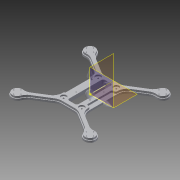
# Autodesk Inventor part: base
Saved by Autodesk Inventor 2013 (Build 170138000, 138)
## iProperties
Created: 2013-06-25
Part Number: base
Material: Aluminum 6061
Document SubType Name: Modeling
Designer: Piotr
Density: 2.71 g/cm^3
Mass: 149.971 g
Surface Area: 272.178 cm^2
Volume: 55.3399 cm^3
Author: Piotr
Autodesk Inventor part; units mm, degrees
ref_plane "YZ Plane" through (0, 0, 0) normal (1, 0, 0) x (0, 1, 0)
ref_plane "XZ Plane" through (0, 0, 0) normal (0, 1, 0) x (-1, 0, 0)
ref_plane "XY Plane" through (0, 0, 0) normal (0, 0, 1) x (1, 0, 0)
sketch "Sketch3" plane through (0, 0, 0) normal (0, 0, 1) x (1, 0, 0)
  line L0 (0, 49) -> (20.5112, 49)
  line L1 (30, 43.117) -> (30, 0)
  line L2 (30, 49) -> (80, 80) construction
  line L3 (30, 43.117) -> (72.8978, 69.7136)
  line L4 (20.5112, 49) -> (67.6284, 78.2127)
  circle A0 centre (80, 80) radius 12.5 construction
  arc A1 (72.8978, 69.7136) -> (67.6284, 78.2127) centre (80, 80) ccw
  line L5 (0, 136.0947) -> (0, -136.0947) construction
  line L6 (-136.0947, 0) -> (136.0947, 0) construction
  line L7 (0, 49) -> (-20.5112, 49)
  line L8 (-30, 43.117) -> (-30, 0)
  line L9 (-30, 43.117) -> (-72.8978, 69.7136)
  line L10 (-20.5112, 49) -> (-67.6284, 78.2127)
  arc A2 (-67.6284, 78.2127) -> (-72.8978, 69.7136) centre (-80, 80) ccw
  line L11 (0, -49) -> (20.5112, -49)
  line L12 (30, -43.117) -> (30, 0)
  line L13 (30, -43.117) -> (72.8978, -69.7136)
  line L14 (20.5112, -49) -> (67.6284, -78.2127)
  arc A3 (67.6284, -78.2127) -> (72.8978, -69.7136) centre (80, -80) ccw
  line L15 (-30, -43.117) -> (-72.8978, -69.7136)
  line L16 (-20.5112, -49) -> (-67.6284, -78.2127)
  line L17 (0, -49) -> (-20.5112, -49)
  line L18 (-30, -43.117) -> (-30, 0)
  arc A4 (-72.8978, -69.7136) -> (-67.6284, -78.2127) centre (-80, -80) ccw
  point P0 (0, 0)
  dimension "d13" = 80
  dimension "d14" = 80
  dimension "d15" = 5
  dimension "d16" = 5
  dimension "d17" = 25
  dimension "d18" = 30
  dimension "d19" = 49
  constraints: 34 end point, 17 symmetric about line, 10 point on circle, 5 centre point, 2 horizontal alignment, 2 parallel, 2 vertical alignment, 1 coincident, 1 concentric, 1 horizontal, 1 perpendicular, 3 other
  measures "d13" horizontal distance of L2.end point (0, 0)
  measures "d14" horizontal distance of point (0, 0) L2.end
  measures "d15" distance between parallel lines of L3 L2
  measures "d16" distance between parallel lines of L2 L4
  measures "d17" diameter of A0
  measures "d18" horizontal distance of point (0, 0) L2.start
  measures "d19" vertical distance of point (0, 0) L2.start
extrude "Extrusion2" add sketch "Sketch3" along normal blind 4
fillet "Fillet1" radius 20 8 edges at (30, 43.117, 2) (30, -43.117, 2) (-30, 43.117, 2) (20.5112, -49, 2) (-30, -43.117, 2) (20.5112, 49, 2) (-20.5112, 49, 2) (-20.5112, -49, 2)
fillet "Fillet2" radius 20 8 edges at (72.8978, 69.7136, 2) (-67.6284, -78.2127, 2) (-72.8978, 69.7136, 2) (67.6284, -78.2127, 2) (72.8978, -69.7136, 2) (67.6284, 78.2127, 2) (-67.6284, 78.2127, 2) (-72.8978, -69.7136, 2)
sketch "Sketch4" plane through (0, 0, 4) normal (0, 0, 1) x (1, 0, 0)
  line L0 (14.8143, 49) -> (-14.8143, 49) projected
  arc A0 (-25.3531, 52.0019) -> (-14.8143, 49) centre (-14.8143, 69) ccw projected
  line L1 (-25.3531, 52.0019) -> (-59.7157, 73.3068) projected
  arc A1 (-68.145, 83.9634) -> (-59.7157, 73.3068) centre (-49.177, 90.3048) ccw projected
  arc A2 (-68.145, 83.9634) -> (-78.2784, 67.6191) centre (-80, 80) ccw projected
  arc A3 (-64.9851, 64.8078) -> (-78.2784, 67.6191) centre (-75.5239, 47.8097) ccw projected
  line L2 (-64.9851, 64.8078) -> (-39.4612, 48.9829) projected
  arc A4 (-30, 31.9849) -> (-39.4612, 48.9829) centre (-50, 31.9849) ccw projected
  line L3 (-30, 31.9849) -> (-30, -31.9849) projected
  arc A5 (-39.4612, -48.9829) -> (-30, -31.9849) centre (-50, -31.9849) ccw projected
  line L4 (-39.4612, -48.9829) -> (-64.9851, -64.8078) projected
  arc A6 (-78.2784, -67.6191) -> (-64.9851, -64.8078) centre (-75.5239, -47.8097) ccw projected
  arc A7 (-78.2784, -67.6191) -> (-68.145, -83.9634) centre (-80, -80) ccw projected
  arc A8 (-59.7157, -73.3068) -> (-68.145, -83.9634) centre (-49.177, -90.3048) ccw projected
  line L5 (-59.7157, -73.3068) -> (-25.3531, -52.0019) projected
  arc A9 (-14.8143, -49) -> (-25.3531, -52.0019) centre (-14.8143, -69) ccw projected
  line L6 (-14.8143, -49) -> (14.8143, -49) projected
  arc A10 (25.3531, -52.0019) -> (14.8143, -49) centre (14.8143, -69) ccw projected
  line L7 (25.3531, -52.0019) -> (59.7157, -73.3068) projected
  arc A11 (68.145, -83.9634) -> (59.7157, -73.3068) centre (49.177, -90.3048) ccw projected
  arc A12 (68.145, -83.9634) -> (78.2784, -67.6191) centre (80, -80) ccw projected
  arc A13 (64.9851, -64.8078) -> (78.2784, -67.6191) centre (75.5239, -47.8097) ccw projected
  line L8 (64.9851, -64.8078) -> (39.4612, -48.9829) projected
  arc A14 (30, -31.9849) -> (39.4612, -48.9829) centre (50, -31.9849) ccw projected
  line L9 (30, -31.9849) -> (30, 31.9849) projected
  arc A15 (39.4612, 48.9829) -> (30, 31.9849) centre (50, 31.9849) ccw projected
  line L10 (39.4612, 48.9829) -> (64.9851, 64.8078) projected
  arc A16 (78.2784, 67.6191) -> (64.9851, 64.8078) centre (75.5239, 47.8097) ccw projected
  arc A17 (78.2784, 67.6191) -> (68.145, 83.9634) centre (80, 80) ccw projected
  arc A18 (59.7157, 73.3068) -> (68.145, 83.9634) centre (49.177, 90.3048) ccw projected
  line L11 (59.7157, 73.3068) -> (25.3531, 52.0019) projected
  arc A19 (14.8143, 49) -> (25.3531, 52.0019) centre (14.8143, 69) ccw projected
  line L12 (-14.8143, 47.5) -> (14.8143, 47.5)
  arc A20 (14.8143, 47.5) -> (26.1435, 50.7271) centre (14.8143, 69) ccw
  line L13 (26.1435, 50.7271) -> (60.5062, 72.0319)
  arc A21 (60.5062, 72.0319) -> (69.5676, 83.4878) centre (49.177, 90.3048) ccw
  arc A22 (78.485, 69.1048) -> (69.5676, 83.4878) centre (80, 80) ccw
  arc A23 (78.485, 69.1048) -> (64.1947, 66.0826) centre (75.5239, 47.8097) ccw
  line L14 (64.1947, 66.0826) -> (38.6708, 50.2578)
  arc A24 (38.6708, 50.2578) -> (28.5, 31.9849) centre (50, 31.9849) ccw
  line L15 (28.5, 31.9849) -> (28.5, -31.9849)
  arc A25 (28.5, -31.9849) -> (38.6708, -50.2578) centre (50, -31.9849) ccw
  line L16 (38.6708, -50.2578) -> (64.1947, -66.0826)
  arc A26 (64.1947, -66.0826) -> (78.485, -69.1048) centre (75.5239, -47.8097) ccw
  arc A27 (69.5676, -83.4878) -> (78.485, -69.1048) centre (80, -80) ccw
  arc A28 (69.5676, -83.4878) -> (60.5062, -72.0319) centre (49.177, -90.3048) ccw
  line L17 (60.5062, -72.0319) -> (26.1435, -50.7271)
  arc A29 (26.1435, -50.7271) -> (14.8143, -47.5) centre (14.8143, -69) ccw
  line L18 (14.8143, -47.5) -> (-14.8143, -47.5)
  arc A30 (-14.8143, -47.5) -> (-26.1435, -50.7271) centre (-14.8143, -69) ccw
  line L19 (-26.1435, -50.7271) -> (-60.5062, -72.0319)
  arc A31 (-60.5062, -72.0319) -> (-69.5676, -83.4878) centre (-49.177, -90.3048) ccw
  arc A32 (-78.485, -69.1048) -> (-69.5676, -83.4878) centre (-80, -80) ccw
  arc A33 (-78.485, -69.1048) -> (-64.1947, -66.0826) centre (-75.5239, -47.8097) ccw
  line L20 (-64.1947, -66.0826) -> (-38.6708, -50.2578)
  arc A34 (-38.6708, -50.2578) -> (-28.5, -31.9849) centre (-50, -31.9849) ccw
  line L21 (-28.5, -31.9849) -> (-28.5, 31.9849)
  arc A35 (-28.5, 31.9849) -> (-38.6708, 50.2578) centre (-50, 31.9849) ccw
  line L22 (-38.6708, 50.2578) -> (-64.1947, 66.0826)
  arc A36 (-64.1947, 66.0826) -> (-78.485, 69.1048) centre (-75.5239, 47.8097) ccw
  arc A37 (-69.5676, 83.4878) -> (-78.485, 69.1048) centre (-80, 80) ccw
  arc A38 (-69.5676, 83.4878) -> (-60.5062, 72.0319) centre (-49.177, 90.3048) ccw
  line L23 (-60.5062, 72.0319) -> (-26.1435, 50.7271)
  arc A39 (-26.1435, 50.7271) -> (-14.8143, 47.5) centre (-14.8143, 69) ccw
  point P0 (0, 0)
  dimension "d24" = 7
  constraints: 40 point on circle, 24 end point, 20 centre point, 31 other
  measures "d24" distance between parallel lines of L23 L22
extrude "Extrusion3" add sketch "Sketch4" along normal blind 4 contours L12 A20 L13 A21 A22 A23 L14 A24 L15 A25 L16 A26 A27 A28 L17 A29 L18 A30 L19 A31 A32 A33 L20 A34 L21 A35 L22 A36 A37 A38 L23 A39
sketch "Sketch5" plane through (0, 0, 0) normal (0, 0, -1) x (-1, 0, 0)
  line L0 (-129.5, 0) -> (129.5, 0) projected
  line L1 (0, -129.5) -> (0, 129.5) projected
  point P0 (0, 0)
  point P1 (-15.25, -15.25)
  point P2 (15.25, -15.25)
  point P3 (15.25, 15.25)
  point P4 (-15.25, 15.25)
  dimension "d28" = 30.5
  dimension "d30" = 30.5
  constraints: 2 horizontal alignment, 2 symmetric about line, 2 vertical alignment
  measures "d28" distance of point (15.25, -15.25) point (15.25, 15.25)
  measures "d30" distance of point (-15.25, 15.25) point (15.25, 15.25)
hole "Hole1" at (15.25, -15.25, 0) at (-15.25, -15.25, 0) at (-15.25, 15.25, 0) at (15.25, 15.25, 0) direction (0, 0, 1) diameter 2.1 end through all
sketch "Sketch6" plane through (0, 0, 8) normal (0, 0, 1) x (1, 0, 0)
  point P0 (0, 0)
  point P1 (-20, -38)
  dimension "d58" = 20
  dimension "d59" = 38
  measures "d58" horizontal distance of point (0, 0) point (-20, -38)
  measures "d59" vertical distance of point (0, 0) point (-20, -38)
hole "Hole2" at (-20, -38, 8) direction (0, 0, -1) diameter 12 depth 3
hole "Hole3" at (-20, -38, 5) direction (0, 0, -1) diameter 3.1 end through all
mirror "Mirror1" about plane through (0, 0, 0) normal (1, 0, 0) of "Hole2", "Hole3"
mirror "Mirror2" about plane through (0, 0, 0) normal (0, 1, 0) of "Hole2", "Hole3", "Mirror1"
sketch "Sketch8" plane through (0, 0, 0) normal (0, 0, -1) x (-1, 0, 0)
  arc A0 (78.2784, 67.6191) -> (68.145, 83.9634) centre (80, 80) ccw projected
  point P0 (0, 0)
  point P1 (80, 88)
  point P2 (72, 80)
  point P3 (80, 72)
  point P4 (88, 80)
  dimension "d60" = 8
  dimension "d63" = 360
  constraints: 1 vertical alignment, 5 other
  measures "d60" distance of A0.centre point (80, 88)
hole "Hole4" at (-80, 88, 0) at (-72, 80, 0) at (-80, 72, 0) at (-88, 80, 0) direction (0, 0, 1) diameter 2.1 end through all
mirror "Mirror3" about plane through (0, 0, 0) normal (0, 1, 0) of "Hole4"
mirror "Mirror4" about plane through (0, 0, 0) normal (1, 0, 0) of "Hole4", "Mirror3"
sketch "Sketch9" plane through (0, 0, 0) normal (0, 0, -1) x (-1, 0, 0)
  circle A0 centre (-80, -72) radius 1.05 projected
  circle A1 centre (-88, -80) radius 1.05 projected
  circle A2 centre (-72, -80) radius 1.05 projected
  circle A3 centre (-80, -88) radius 1.05 projected
  circle A4 centre (-80, 72) radius 1.05 projected
  circle A5 centre (-88, 80) radius 1.05 projected
  circle A6 centre (-72, 80) radius 1.05 projected
  circle A7 centre (-80, 88) radius 1.05 projected
  circle A8 centre (80, -72) radius 1.05 projected
  circle A9 centre (88, -80) radius 1.05 projected
  circle A10 centre (72, -80) radius 1.05 projected
  circle A11 centre (80, -88) radius 1.05 projected
  circle A12 centre (80, 72) radius 1.05 projected
  circle A13 centre (80, 88) radius 1.05 projected
  circle A14 centre (72, 80) radius 1.05 projected
  circle A15 centre (88, 80) radius 1.05 projected
  circle A16 centre (-20, 38) radius 6 projected
  circle A17 centre (20, 38) radius 6 projected
  circle A18 centre (-20, -38) radius 6 projected
  circle A19 centre (20, -38) radius 6 projected
  circle A20 centre (15.25, 15.25) radius 1.05 projected
  circle A21 centre (-15.25, -15.25) radius 1.05 projected
  circle A22 centre (15.25, -15.25) radius 1.05 projected
  circle A23 centre (-15.25, 15.25) radius 1.05 projected
  line L0 (-14.8143, 47.5) -> (14.8143, 47.5) projected
  arc A24 (14.8143, 47.5) -> (26.1435, 50.7271) centre (14.8143, 69) ccw projected
  line L1 (26.1435, 50.7271) -> (60.5062, 72.0319) projected
  arc A25 (60.5062, 72.0319) -> (69.5676, 83.4878) centre (49.177, 90.3048) ccw projected
  arc A26 (78.485, 69.1048) -> (69.5676, 83.4878) centre (80, 80) ccw projected
  arc A27 (78.485, 69.1048) -> (64.1947, 66.0826) centre (75.5239, 47.8097) ccw projected
  line L2 (64.1947, 66.0826) -> (38.6708, 50.2578) projected
  arc A28 (38.6708, 50.2578) -> (28.5, 31.9849) centre (50, 31.9849) ccw projected
  line L3 (28.5, 31.9849) -> (28.5, -31.9849) projected
  arc A29 (28.5, -31.9849) -> (38.6708, -50.2578) centre (50, -31.9849) ccw projected
  line L4 (38.6708, -50.2578) -> (64.1947, -66.0826) projected
  arc A30 (64.1947, -66.0826) -> (78.485, -69.1048) centre (75.5239, -47.8097) ccw projected
  arc A31 (69.5676, -83.4878) -> (78.485, -69.1048) centre (80, -80) ccw projected
  arc A32 (69.5676, -83.4878) -> (60.5062, -72.0319) centre (49.177, -90.3048) ccw projected
  line L5 (60.5062, -72.0319) -> (26.1435, -50.7271) projected
  arc A33 (26.1435, -50.7271) -> (14.8143, -47.5) centre (14.8143, -69) ccw projected
  line L6 (14.8143, -47.5) -> (-14.8143, -47.5) projected
  arc A34 (-14.8143, -47.5) -> (-26.1435, -50.7271) centre (-14.8143, -69) ccw projected
  line L7 (-26.1435, -50.7271) -> (-60.5062, -72.0319) projected
  arc A35 (-60.5062, -72.0319) -> (-69.5676, -83.4878) centre (-49.177, -90.3048) ccw projected
  arc A36 (-78.485, -69.1048) -> (-69.5676, -83.4878) centre (-80, -80) ccw projected
  arc A37 (-78.485, -69.1048) -> (-64.1947, -66.0826) centre (-75.5239, -47.8097) ccw projected
  line L8 (-64.1947, -66.0826) -> (-38.6708, -50.2578) projected
  arc A38 (-38.6708, -50.2578) -> (-28.5, -31.9849) centre (-50, -31.9849) ccw projected
  line L9 (-28.5, -31.9849) -> (-28.5, 31.9849) projected
  arc A39 (-28.5, 31.9849) -> (-38.6708, 50.2578) centre (-50, 31.9849) ccw projected
  line L10 (-38.6708, 50.2578) -> (-64.1947, 66.0826) projected
  arc A40 (-64.1947, 66.0826) -> (-78.485, 69.1048) centre (-75.5239, 47.8097) ccw projected
  arc A41 (-69.5676, 83.4878) -> (-78.485, 69.1048) centre (-80, 80) ccw projected
  arc A42 (-69.5676, 83.4878) -> (-60.5062, 72.0319) centre (-49.177, 90.3048) ccw projected
  line L11 (-60.5062, 72.0319) -> (-26.1435, 50.7271) projected
  arc A43 (-26.1435, 50.7271) -> (-14.8143, 47.5) centre (-14.8143, 69) ccw projected
  line L12 (-10.5, 39.5) -> (10.5, 39.5)
  line L13 (10.5, 39.5) -> (10.5, -39.5)
  line L14 (10.5, -39.5) -> (-10.5, -39.5)
  line L15 (-10.5, -39.5) -> (-10.5, 39.5)
  point P0 (0, 0)
  dimension "d72" = 8
  dimension "d73" = 8
  dimension "d74" = 18
  dimension "d75" = 18
  constraints: 8 end point, 2 parallel, 1 horizontal, 1 perpendicular
  measures "d72" distance between parallel lines of L0 L12
  measures "d73" distance between parallel lines of L6 L14
  measures "d74" distance between parallel lines of L3 L13
  measures "d75" distance between parallel lines of L9 L15
extrude "Extrusion4" cut sketch "Sketch9" against normal blind 11.5 contours L12 L13 L14 L15
fillet "Fillet3" radius 4 4 edges at (10.5, 39.5, 4) (-10.5, 39.5, 4) (10.5, -39.5, 4) (-10.5, -39.5, 4)
sketch "Sketch10" plane through (0, 0, 8) normal (0, 0, 1) x (1, 0, 0)
  line L0 (-10.5, -35.5) -> (-10.5, 35.5) projected
  circle A0 centre (-20, 38) radius 6 projected
  circle A1 centre (-20, -38) radius 6 projected
  line L1 (-28.5, 31.9849) -> (-28.5, -31.9849) projected
  line L2 (-28.5, 28) -> (-20.5, 28)
  line L3 (-20.5, 28) -> (-20.5, -28)
  line L4 (-20.5, -28) -> (-28.5, -28)
  line L5 (-28.5, -28) -> (-28.5, 28)
  point P0 (0, 0)
  dimension "d84" = 10
  dimension "d85" = 10
  dimension "d86" = 10
  constraints: 8 end point, 2 parallel, 1 horizontal, 1 perpendicular, 1 point on line
  measures "d84" distance from line of A0.centre L2
  measures "d85" distance from line of A1.centre L4
  measures "d86" distance between parallel lines of L0 L3
extrude "Extrusion5" cut sketch "Sketch10" against normal blind 4 contours L2 L3 L4 L1
mirror "Mirror5" about plane through (0, 0, 0) normal (1, 0, 0) of "Extrusion5"
fillet "Fillet5" radius 3 8 edges at (20.5, 28, 6) (28.5, 28, 6) (-20.5, 28, 6) (-28.5, 28, 6) (-28.5, -28, 6) (-20.5, -28, 6) (20.5, -28, 6) (28.5, -28, 6)
equation "\"d14\" = d13"
equation "\"d16\" = d15"
equation "\"d30\" = d28"
equation "\"d73\" = d72"
equation "\"d75\" = d74"
equation "\"d85\" = d84"
body "Solid2"
